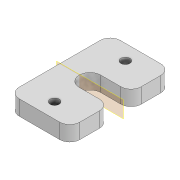
# Autodesk Inventor part: shaft pusher bottom
Saved by Autodesk Inventor 2020 (Build 240168000, 168)
## iProperties
Created: 2020-05-29
Part Number: shaft pusher bottom
Material: Generic
Document SubType Name: Modeling
Designer: mrbeh
Density: 1 g/cm^3
Appearance: Default
Author: mrbeh
Autodesk Inventor part; units mm, degrees
ref_plane "YZ Plane" through (0, 0, 0) normal (1, 0, 0) x (0, 1, 0)
ref_plane "XZ Plane" through (0, 0, 0) normal (0, 1, 0) x (-1, 0, 0)
ref_plane "XY Plane" through (0, 0, 0) normal (0, 0, 1) x (1, 0, 0)
sketch "Sketch1" plane through (0, 0, 0) normal (0, 1, 0) x (-1, 0, 0)
  line L0 (0, 0) -> (24, 0)
  line L1 (24, 0) -> (24, -40)
  line L2 (24, -40) -> (0, -40)
  line L3 (0, -40) -> (0, 0)
  dimension "d0" = 24
  dimension "d1" = 40
  constraints: 8 end point, 2 parallel, 1 horizontal, 1 perpendicular
  measures "d0" distance of L1.end L2.end
  measures "d1" distance of L0.end L1.end
extrude "Extrusion1" add sketch "Sketch1" along normal blind 6
sketch "Sketch2" plane through (0, 6, 0) normal (0, 1, 0) x (1, 0, 0)
  arc A0 (-12, 24.25) -> (-12, 15.75) centre (-12, 20) ccw
  line L0 (-12, 15.75) -> (0, 15.75)
  line L1 (-12, 24.25) -> (0, 24.25)
  line L2 (0, 24.25) -> (0, 15.75)
  line L3 (0, 0) -> (0, 40) projected
  dimension "d4" = 8.5
  constraints: 6 end point, 2 horizontal, 2 point on circle, 1 centre point, 1 collinear
  measures "d4" diameter of A0
extrude "Extrusion2" cut sketch "Sketch2" against normal blind 6
sketch "Sketch3" plane through (0, 6, 0) normal (0, 1, 0) x (1, 0, 0)
  circle A0 centre (-12, 6) radius 1.8
  point P0 (0, 0)
  dimension "d7" = 3.6
  constraints: 1 centre point
  measures "d7" diameter of A0
extrude "Extrusion3" cut sketch "Sketch3" against normal blind 6
ref_plane "Work Plane1" through (-24, 0, -20) normal (0, 0, 1) x (1, 0, 0)
mirror "Mirror1" about plane through (-24, 0, -20) normal (0, 0, 1) of "Extrusion3"
sketch "Sketch4" plane through (0, 0, 0) normal (0, -1, 0) x (1, 0, 0)
  circle A0 centre (-12, -6) radius 1.8 projected
  circle A1 centre (-12, -6) radius 2.9
  point P0 (0, 0)
  dimension "d11" = 5.8
  constraints: 1 centre point, 1 coincident
  measures "d11" diameter of A1
extrude "Extrusion4" cut sketch "Sketch4" against normal blind 3
mirror "Mirror2" about plane through (-24, 0, -20) normal (0, 0, 1) of "Extrusion4"
fillet "Fillet1" radius 4 6 edges at (-24, 3, -40) (0, 3, 0) (-24, 3, 0) (0, 3, -40) (0, 3, -24.25) (0, 3, -15.75)
body "Solid1"
